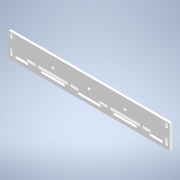
# Autodesk Inventor part: case top front
Saved by Autodesk Inventor 2022 (Build 260153000, 153)
## iProperties
Created: 2021-05-28
Part Number: case top front
Material: ABS Plastic
Document SubType Name: Modeling
Designer: benka
Density: 1.06 g/cm^3
Appearance: Smooth - White
Author: benka
Autodesk Inventor part; units mm, degrees
ref_plane "YZ Plane" through (0, 0, 0) normal (1, 0, 0) x (0, 1, 0)
ref_plane "XZ Plane" through (0, 0, 0) normal (0, 1, 0) x (-1, 0, 0)
ref_plane "XY Plane" through (0, 0, 0) normal (0, 0, 1) x (1, 0, 0)
sketch "Sketch1" plane through (0, 0, 0) normal (0, 0, 1) x (1, 0, 0)
  line L0 (57.983, -13.2177) -> (41.983, -13.2177)
  line L1 (41.983, -18.2177) -> (57.983, -18.2177)
  line L2 (-58.017, -13.2177) -> (-42.017, -13.2177)
  line L3 (-42.017, -18.2177) -> (-58.017, -18.2177)
  line L4 (32.983, -13.2177) -> (-33.017, -13.2177)
  line L5 (-33.017, -18.2177) -> (32.983, -18.2177)
  arc A0 (34.983, -15.2177) -> (32.983, -13.2177) centre (32.983, -15.2177) ccw
  arc A1 (-35.017, -16.2177) -> (-33.017, -18.2177) centre (-33.017, -16.2177) ccw
  arc A2 (-33.017, -13.2177) -> (-35.017, -15.2177) centre (-33.017, -15.2177) ccw
  arc A3 (-40.017, -15.2177) -> (-42.017, -13.2177) centre (-42.017, -15.2177) ccw
  arc A4 (-42.017, -18.2177) -> (-40.017, -16.2177) centre (-42.017, -16.2177) ccw
  arc A5 (-60.017, -16.2177) -> (-58.017, -18.2177) centre (-58.017, -16.2177) ccw
  arc A6 (-58.017, -13.2177) -> (-60.017, -15.2177) centre (-58.017, -15.2177) ccw
  arc A7 (39.983, -16.2177) -> (41.983, -18.2177) centre (41.983, -16.2177) ccw
  arc A8 (41.983, -13.2177) -> (39.983, -15.2177) centre (41.983, -15.2177) ccw
  arc A9 (59.983, -15.2177) -> (57.983, -13.2177) centre (57.983, -15.2177) ccw
  arc A10 (57.983, -18.2177) -> (59.983, -16.2177) centre (57.983, -16.2177) ccw
  arc A11 (32.983, -18.2177) -> (34.983, -16.2177) centre (32.983, -16.2177) ccw
  line L6 (59.983, -15.2177) -> (39.983, -15.2177)
  line L7 (39.983, -16.2177) -> (59.983, -16.2177)
  line L8 (34.983, -15.2177) -> (-35.017, -15.2177)
  line L9 (-35.017, -16.2177) -> (34.983, -16.2177)
  line L10 (-40.017, -15.2177) -> (-60.017, -15.2177)
  line L11 (-60.017, -16.2177) -> (-40.017, -16.2177)
  line L12 (-57.517, -25.0011) -> (-110.517, -25.0011) projected
  line L13 (-110.517, -25.0011) -> (-110.517, -20.0011) projected
  line L14 (-57.517, -20.0011) -> (-110.517, -20.0011) projected
  line L15 (-57.517, -25.0011) -> (-57.517, -20.0011) projected
  line L16 (-140.517, -25.0011) -> (-195.517, -25.0011) projected
  line L17 (-195.517, -25.0011) -> (-195.517, -20.0011) projected
  line L18 (-140.517, -20.0011) -> (-195.517, -20.0011) projected
  line L19 (-140.517, -25.0011) -> (-140.517, -20.0011) projected
  line L20 (-225.517, -25.0011) -> (-255.517, -25.0011) projected
  line L21 (-255.517, -25.0011) -> (-255.517, -20.0011) projected
  line L22 (-225.517, -20.0011) -> (-255.517, -20.0011) projected
  line L23 (-225.517, -25.0011) -> (-225.517, -20.0011) projected
  line L24 (-272.017, -33.0013) -> (103.983, -33.0013)
  line L25 (98.983, 19.9989) -> (98.983, 9.9974) projected
  line L26 (98.983, 9.9974) -> (93.983, 9.9974) projected
  line L27 (93.983, 19.9989) -> (93.983, 9.9974) projected
  line L28 (98.983, 19.9989) -> (93.983, 19.9989) projected
  line L29 (98.983, -10.0026) -> (98.983, -25.0018) projected
  line L30 (98.983, -25.0018) -> (93.983, -25.0018) projected
  line L31 (93.983, -10.0026) -> (93.983, -25.0018) projected
  line L32 (98.983, -10.0026) -> (93.983, -10.0026) projected
  line L33 (-262.017, -10.0026) -> (-262.017, -25.0018) projected
  line L34 (-262.017, -25.0018) -> (-267.017, -25.0018) projected
  line L35 (-267.017, -10.0026) -> (-267.017, -25.0018) projected
  line L36 (-262.017, -10.0026) -> (-267.017, -10.0026) projected
  line L37 (-262.017, 19.9989) -> (-262.017, 9.9974) projected
  line L38 (-262.017, 9.9974) -> (-267.017, 9.9974) projected
  line L39 (-267.017, 19.9989) -> (-267.017, 9.9974) projected
  line L40 (-262.017, 19.9989) -> (-267.017, 19.9989) projected
  line L41 (-110.017, -13.2177) -> (-126.017, -13.2177)
  line L42 (-126.017, -18.2177) -> (-110.017, -18.2177)
  line L43 (-226.017, -13.2177) -> (-210.017, -13.2177)
  line L44 (-210.017, -18.2177) -> (-226.017, -18.2177)
  line L45 (-135.017, -13.2177) -> (-201.017, -13.2177)
  line L46 (-201.017, -18.2177) -> (-135.017, -18.2177)
  arc A12 (-133.017, -15.2177) -> (-135.017, -13.2177) centre (-135.017, -15.2177) ccw
  arc A13 (-203.017, -16.2177) -> (-201.017, -18.2177) centre (-201.017, -16.2177) ccw
  arc A14 (-201.017, -13.2177) -> (-203.017, -15.2177) centre (-201.017, -15.2177) ccw
  arc A15 (-208.017, -15.2177) -> (-210.017, -13.2177) centre (-210.017, -15.2177) ccw
  arc A16 (-210.017, -18.2177) -> (-208.017, -16.2177) centre (-210.017, -16.2177) ccw
  arc A17 (-228.017, -16.2177) -> (-226.017, -18.2177) centre (-226.017, -16.2177) ccw
  arc A18 (-226.017, -13.2177) -> (-228.017, -15.2177) centre (-226.017, -15.2177) ccw
  arc A19 (-128.017, -16.2177) -> (-126.017, -18.2177) centre (-126.017, -16.2177) ccw
  arc A20 (-126.017, -13.2177) -> (-128.017, -15.2177) centre (-126.017, -15.2177) ccw
  arc A21 (-108.017, -15.2177) -> (-110.017, -13.2177) centre (-110.017, -15.2177) ccw
  arc A22 (-110.017, -18.2177) -> (-108.017, -16.2177) centre (-110.017, -16.2177) ccw
  arc A23 (-135.017, -18.2177) -> (-133.017, -16.2177) centre (-135.017, -16.2177) ccw
  line L47 (-108.017, -15.2177) -> (-128.017, -15.2177)
  line L48 (-128.017, -16.2177) -> (-108.017, -16.2177)
  line L49 (-133.017, -15.2177) -> (-203.017, -15.2177)
  line L50 (-203.017, -16.2177) -> (-133.017, -16.2177)
  line L51 (-208.017, -15.2177) -> (-228.017, -15.2177)
  line L52 (-228.017, -16.2177) -> (-208.017, -16.2177)
  line L53 (87.483, -25.0011) -> (57.483, -25.0011) projected
  line L54 (57.483, -25.0011) -> (57.483, -20.0011) projected
  line L55 (87.483, -20.0011) -> (57.483, -20.0011) projected
  line L56 (87.483, -25.0011) -> (87.483, -20.0011) projected
  line L57 (27.483, -25.0011) -> (-27.517, -25.0011) projected
  line L58 (-27.517, -25.0011) -> (-27.517, -20.0011) projected
  line L59 (27.483, -20.0011) -> (-27.517, -20.0011) projected
  line L60 (27.483, -25.0011) -> (27.483, -20.0011) projected
  circle A24 centre (-84.017, -1.0005) radius 3
  line L61 (103.983, 20.9995) -> (103.983, -33.0013)
  circle A25 centre (-0.017, -1.0005) radius 3
  line L62 (-272.017, 20.9995) -> (-272.017, -33.0013)
  circle A26 centre (-168.017, -1.0005) radius 3
  line L63 (101.983, 22.9995) -> (-270.017, 22.9995)
  arc A27 (103.983, 20.9995) -> (101.983, 22.9995) centre (101.983, 20.9995) ccw
  arc A28 (-270.017, 22.9995) -> (-272.017, 20.9995) centre (-270.017, 20.9995) ccw
  point P0 (103.983, 22.9995)
  point P1 (59.983, -13.2177)
  point P2 (59.983, -18.2177)
  point P3 (59.983, -16.2177)
  point P4 (-108.017, -13.2177)
  point P5 (-108.017, -18.2177)
  point P6 (-272.017, 22.9995)
  dimension "d17" = 5
  dimension "d27" = 2
  dimension "d36" = 5
  dimension "d37" = 2
  dimension "d39" = 6
  dimension "d40" = 6
  dimension "d42" = 188
  dimension "d44" = 376
  dimension "d45" = 188
  dimension "d46" = 84
  dimension "d47" = 6
  dimension "d48" = 84
  dimension "d50" = 2
  constraints: 56 end point, 54 point on circle, 29 centre point, 28 tangent, 23 equal radius, 20 point on line, 14 horizontal, 12 parallel, 8 collinear, 1 perpendicular, 1 vertical
  measures "d17" distance of point (59.983, -18.218) point (59.983, -13.218)
  measures "d27" radius of A0
  measures "d36" distance of point (-108.017, -18.218) point (-108.017, -13.218)
  measures "d37" radius of A12
  measures "d39" diameter of A24
  measures "d40" diameter of A25
  measures "d42" distance from line of L61 A24.centre
  measures "d44" distance between parallel lines of L62 L61
  measures "d45" distance from line of L62 A24.centre
  measures "d46" distance of A25.centre A24.centre
  measures "d47" diameter of A26
  measures "d48" distance of A26.centre A24.centre
  measures "d50" radius of A27
extrude "Extrusion1" add sketch "Sketch1" along normal blind 5
body "Solid1"
